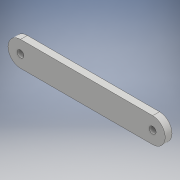
# Autodesk Inventor part: biela
Saved by Autodesk Inventor 2018 (Build 220112000, 112)
## iProperties
Created: 2020-03-10
Part Number: biela
Material: Genérico
Document SubType Name: Modeling
Designer: sala.ceri
Density: 1 g/cm^3
Appearance: Valor por defecto
Author: sala.ceri
Autodesk Inventor part; units mm, degrees
ref_plane "YZ Plane" through (0, 0, 0) normal (1, 0, 0) x (0, 1, 0)
ref_plane "XZ Plane" through (0, 0, 0) normal (0, 1, 0) x (-1, 0, 0)
ref_plane "XY Plane" through (0, 0, 0) normal (0, 0, 1) x (1, 0, 0)
sketch "Boceto1" plane through (0, 0, 0) normal (0, 1, 0) x (-1, 0, 0)
  arc A0 (119.9994, -35.5039) -> (120.0001, -24.5039) centre (119.9998, -30.0039) ccw
  arc A1 (62, -24.5) -> (61.9993, -35.5) centre (61.9996, -30) ccw
  line L0 (62, -24.5) -> (120.0001, -24.5039)
  line L1 (119.9994, -35.5039) -> (61.9993, -35.5)
  circle A2 centre (119.9998, -30.0039) radius 1.5
  circle A3 centre (61.9996, -30) radius 1.5
  point P0 (124.9998, -30.0039)
  point P1 (119.9998, -25.0039)
  dimension "d172" = 3
  dimension "d173" = 3
  constraints: 4 centre point, 4 end point, 4 point on circle, 2 coincident, 1 parallel, 1 tangent
  measures "d172" diameter of A2
  measures "d173" diameter of A3
extrude "Extrusión1" add sketch "Boceto1" along normal blind 3
